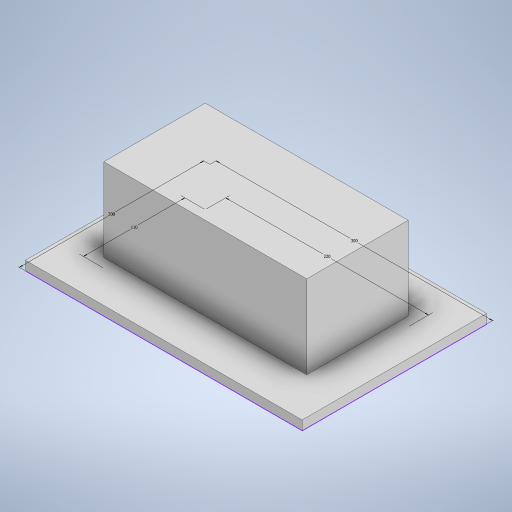
# Autodesk Inventor part: Part1
Saved by Autodesk Inventor 2024 (Build 280153000, 153)
## iProperties
Created: 2023-07-03
Part Number: Part1
Material: Generic
Document SubType Name: Modeling
Designer: janro
Density: 1 g/cm^3
Appearance: Default
Author: janro
Autodesk Inventor part; units mm, degrees
ref_plane "YZ Plane" through (0, 0, 0) normal (1, 0, 0) x (0, 1, 0)
ref_plane "XZ Plane" through (0, 0, 0) normal (0, 1, 0) x (-1, 0, 0)
ref_plane "XY Plane" through (0, 0, 0) normal (0, 0, 1) x (1, 0, 0)
sketch "Sketch1" plane through (0, 0, 0) normal (0, 1, 0) x (-1, 0, 0)
  line L0 (-150, 100) -> (150, 100)
  line L1 (150, 100) -> (150, -100)
  line L2 (150, -100) -> (-150, -100)
  line L3 (-150, -100) -> (-150, 100)
  line L4 (-110, 55) -> (110, 55)
  line L5 (110, 55) -> (110, -55)
  line L6 (110, -55) -> (-110, -55)
  line L7 (-110, -55) -> (-110, 55)
  line L8 (-110, 55) -> (110, -55) construction
  line L9 (110, 55) -> (-110, -55) construction
  point P0 (0, 0)
  dimension "d0" = 300
  dimension "d1" = 200
  dimension "d3" = 220
  dimension "d4" = 110
  constraints: 20 end point, 4 parallel, 2 horizontal, 2 midpoint, 2 perpendicular
  measures "d0" distance of L1.end L2.end
  measures "d1" distance of L0.end L1.end
  measures "d3" distance of L5.end L6.end
  measures "d4" distance of L4.end L5.end
extrude "Extrusion1" add sketch "Sketch1" along normal blind 10
extrude "Extrusion2" add sketch "Sketch1" along normal blind 100 contours L4 L5 L6 L7
extrude "Extrusion3" add sketch "Sketch1" against normal blind 30 contours L4 L5 L6 L7
body "Solid1"
